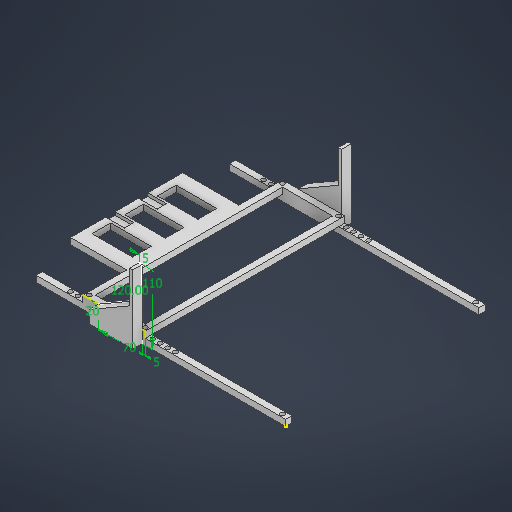
# Autodesk Inventor part: Pedal Box Mount V1
Saved by Autodesk Inventor 2027 (Build 310192000, 192)
## iProperties
Created: 2026-07-08
Part Number: Pedal Box Mount V1
Material: Generic
Document SubType Name: Modeling
Designer: W Ahmad
Density: 1 g/cm^3
Appearance: Default
Author: W Ahmad
Autodesk Inventor part; units mm, degrees
ref_plane "YZ Plane" through (0, 0, 0) normal (1, 0, 0) x (0, 1, 0)
ref_plane "XZ Plane" through (0, 0, 0) normal (0, 1, 0) x (-1, 0, 0)
ref_plane "XY Plane" through (0, 0, 0) normal (0, 0, 1) x (1, 0, 0)
sketch "Sketch1" plane through (0, 0, 0) normal (0, 1, 0) x (-1, 0, 0)
  line L0 (400, 160) -> (0, 160)
  line L1 (0, 160) -> (0, 150)
  line L2 (0, 150) -> (400, 150)
  line L3 (400, 150) -> (400, 160)
  line L4 (400, -150) -> (0, -150)
  line L5 (0, -150) -> (0, -160)
  line L6 (0, -160) -> (400, -160)
  line L7 (400, -160) -> (400, -150)
  line L8 (0, 150) -> (0, 0) construction
  line L9 (0, 0) -> (200, 0) construction
  circle A0 centre (350, 155) radius 3.5
  circle A1 centre (350, -155) radius 3.5
  circle A2 centre (338, 155) radius 3.5
  circle A3 centre (338, -155) radius 3.5
  circle A4 centre (326, 155) radius 3.5
  circle A5 centre (326, -155) radius 3.5
  circle A6 centre (314, 155) radius 3.5
  circle A7 centre (314, -155) radius 3.5
  circle A8 centre (302, 155) radius 3.5
  circle A9 centre (302, -155) radius 3.5
  circle A10 centre (290, 155) radius 3.5
  circle A11 centre (290, -155) radius 3.5
  circle A12 centre (278, 155) radius 3.5
  circle A13 centre (278, -155) radius 3.5
  circle A14 centre (266, 155) radius 3.5
  circle A15 centre (266, -155) radius 3.5
  circle A16 centre (254, 155) radius 3.5
  circle A17 centre (254, -155) radius 3.5
  circle A18 centre (242, 155) radius 3.5
  circle A19 centre (242, -155) radius 3.5
  circle A20 centre (230, 155) radius 3.5
  circle A21 centre (230, -155) radius 3.5
  circle A22 centre (218, 155) radius 3.5
  circle A23 centre (218, -155) radius 3.5
  circle A24 centre (206, 155) radius 3.5
  circle A25 centre (206, -155) radius 3.5
  circle A26 centre (194, 155) radius 3.5
  circle A27 centre (194, -155) radius 3.5
  circle A28 centre (182, 155) radius 3.5
  circle A29 centre (182, -155) radius 3.5
  circle A30 centre (10, 155) radius 3.5
  circle A31 centre (10, -155) radius 3.5
  point P0 (400, 155)
  point P1 (400, -155)
  point P2 (0, -155)
  point P3 (0, 155)
  dimension "d0" = 10
  dimension "d1" = 400
  dimension "d2" = 300
  dimension "d3" = 150
  dimension "d4" = 200
  dimension "d5" = 50
  dimension "d6" = 7
  dimension "d7" = 7
  dimension "d8" = 50
  dimension "d11" = 12
  dimension "d16" = 7
  dimension "d17" = 10
  dimension "d18" = 10
  dimension "d19" = 7
  constraints: 32 centre point, 20 end point, 4 horizontal alignment, 4 midpoint, 4 parallel, 3 horizontal, 3 perpendicular, 2 point on line, 1 coincident, 1 collinear, 1 vertical, 56 other
  measures "d0" distance of L2.end L0.start
  measures "d1" distance of L0.start L0.end
  measures "d2" distance between parallel lines of L4 L2
  measures "d3" distance of L1.end L8.end
  measures "d4" distance of L8.end L9.end
  measures "d5" distance from line of L3 A0.centre
  measures "d6" diameter of A0
  measures "d7" diameter of A1
  measures "d8" distance from line of A1.centre L7
  measures "d11" distance of A0.centre A2.centre
  measures "d16" diameter of A31
  measures "d17" distance from line of L5 A31.centre
  measures "d18" distance from line of L1 A30.centre
  measures "d19" diameter of A30
extrude "Extrusion1" add sketch "Sketch1" along normal blind 10
sketch "Sketch2" plane through (0, 10, 0) normal (0, 1, 0) x (1, 0, 0)
  line L0 (-325, -160) -> (-225, -160)
  line L1 (-225, -160) -> (-225, 160)
  line L2 (-225, 160) -> (-325, 160)
  line L3 (-325, 160) -> (-325, -160)
  line L4 (0, 160) -> (-400, 160) projected
  line L5 (-400, -160) -> (0, -160) projected
  line L6 (0, -150) -> (-400, -150) projected
  line L7 (-400, 150) -> (0, 150) projected
  line L8 (-315, -150) -> (-235, -150)
  line L9 (-235, -150) -> (-235, 150)
  line L10 (-235, 150) -> (-315, 150)
  line L11 (-315, 150) -> (-315, -150)
  line L12 (-325, -90) -> (-415, -90)
  line L13 (-415, -90) -> (-415, 90)
  line L14 (-415, 90) -> (-325, 90)
  line L15 (-325, 90) -> (-325, -90)
  line L16 (-403, -67.5) -> (-338, -67.5)
  line L17 (-338, -67.5) -> (-338, -37.5)
  line L18 (-338, -37.5) -> (-403, -37.5)
  line L19 (-403, -37.5) -> (-403, -67.5)
  line L20 (-403, -15) -> (-338, -15)
  line L21 (-338, -15) -> (-338, 15)
  line L22 (-338, 15) -> (-403, 15)
  line L23 (-403, 15) -> (-403, -15)
  line L24 (-403, 37.5) -> (-338, 37.5)
  line L25 (-338, 37.5) -> (-338, 67.5)
  line L26 (-338, 67.5) -> (-403, 67.5)
  line L27 (-403, 67.5) -> (-403, 37.5)
  circle A0 centre (-320, -155) radius 3.5
  line L28 (0, -160) -> (0, -150) projected
  circle A1 centre (-320, 155) radius 3.5
  line L29 (-400, 160) -> (-400, 150) projected
  circle A2 centre (-230, -155) radius 3.5
  circle A3 centre (-230, 155) radius 3.5
  point P0 (0, 0)
  point P1 (-325, 0)
  point P2 (0, -155)
  point P3 (-400, 155)
  dimension "d22" = 0
  dimension "d23" = 0
  dimension "d25" = 10
  dimension "d26" = 10
  dimension "d27" = 80
  dimension "d28" = 225
  dimension "d31" = 180
  dimension "d33" = 60
  dimension "d34" = 90
  dimension "d35" = 30
  dimension "d36" = 30
  dimension "d37" = 30
  dimension "d38" = 65
  dimension "d41" = 12
  dimension "d42" = 22.5
  dimension "d43" = 22.5
  dimension "d44" = 22.5
  dimension "d48" = 5
  dimension "d49" = 7
  dimension "d50" = 5
  dimension "d51" = 7
  dimension "d54" = 90
  constraints: 48 end point, 12 parallel, 7 horizontal, 6 perpendicular, 5 point on line, 4 centre point, 3 midpoint, 2 collinear, 2 horizontal alignment, 4 other
  measures "d22" distance between parallel lines of L4 L2
  measures "d23" distance between parallel lines of L5 L0
  measures "d25" distance between parallel lines of L11 L3
  measures "d26" distance between parallel lines of L1 L9
  measures "d27" distance of L8.start L8.end
  measures "d28" distance from line of point (0, 0) L1
  measures "d31" distance of L12.end L13.end
  measures "d33" distance between parallel lines of L12 L6
  measures "d34" distance of L13.end L14.end
  measures "d35" distance of L22.end L20.start
  measures "d36" distance of L26.end L24.start
  measures "d37" distance of L18.end L16.start
  measures "d38" distance of L20.start L20.end
  measures "d41" distance between parallel lines of L23 L13
  measures "d42" distance between parallel lines of L14 L26
  measures "d43" distance between parallel lines of L24 L22
  measures "d44" distance between parallel lines of L20 L18
  measures "d48" distance from line of A0.centre L3
  measures "d49" diameter of A0
  measures "d50" distance from line of A1.centre L3
  measures "d51" diameter of A1
  measures "d54" distance of A0.centre A2.centre
extrude "Extrusion3" add sketch "Sketch2" along normal blind 10 contours L3 L6 L1 L0 | L3 L7 L11 L6 | L6 L9 L7 L1 | L12 L13 L14 L3 | L7 L3 L2 L1
sketch "Sketch3" plane through (0, 20, 0) normal (0, 1, 0) x (1, 0, 0)
  line L0 (-415, 90) -> (-415, -90) projected
  line L1 (-415, -33.5) -> (-385, -33.5)
  line L2 (-385, -33.5) -> (-385, -18.5)
  line L3 (-385, -18.5) -> (-415, -18.5)
  line L4 (-415, -18.5) -> (-415, -33.5)
  line L5 (-415, 19) -> (-385, 19)
  line L6 (-385, 19) -> (-385, 34)
  line L7 (-385, 34) -> (-415, 34)
  line L8 (-415, 34) -> (-415, 19)
  line L9 (-403, 15) -> (-338, 15) projected
  line L10 (-403, -37.5) -> (-338, -37.5) projected
  point P0 (0, 0)
  dimension "d61" = 0
  dimension "d62" = 30
  dimension "d63" = 15
  dimension "d64" = 15
  dimension "d65" = 4
  dimension "d66" = 4
  constraints: 16 end point, 4 parallel, 2 horizontal, 2 perpendicular, 1 collinear, 1 point on line
  measures "d61" distance between parallel lines of L0 L8
  measures "d62" distance of L1.start L1.end
  measures "d63" distance of L1.end L2.end
  measures "d64" distance of L5.end L6.end
  measures "d65" distance between parallel lines of L5 L9
  measures "d66" distance between parallel lines of L1 L10
extrude "Extrusion4" cut sketch "Sketch3" against normal blind 5
sketch "Sketch4" plane through (-400, 0, 160) normal (0, 0, 1) x (1, 0, 0)
  line L0 (100, 0) -> (170, 0)
  line L1 (170, 0) -> (170, 110)
  line L2 (170, 110) -> (165, 110)
  line L3 (165, 110) -> (165, 57.5278)
  line L4 (100, 0) -> (100, 20)
  line L5 (75, 20) -> (175, 20) projected
  line L6 (165, 57.5278) -> (100, 20)
  line L7 (175, 10) -> (175, 20) projected
  point P0 (400, 0)
  dimension "d69" = 120
  dimension "d70" = 5
  dimension "d71" = 110
  dimension "d72" = 70
  dimension "d73" = 20
  dimension "d74" = 5
  constraints: 12 end point, 3 perpendicular, 1 horizontal, 1 point on line, 1 vertical
  measures "d69" angle of L3 L6
  measures "d70" distance of L1.end L2.end
  measures "d71" distance of L0.end L1.end
  measures "d72" distance of L0.start L0.end
  measures "d73" distance of L0.start L4.end
  measures "d74" distance between parallel lines of L7 L1
extrude "Extrusion5" add sketch "Sketch4" along normal blind 15
sketch "Sketch5" plane through (0, 0, -160) normal (0, 0, -1) x (-1, 0, 0)
  line L0 (300, 0) -> (230, 0) projected
  line L1 (300, 0) -> (230, 0)
  line L2 (230, 0) -> (230, 110)
  line L3 (230, 110) -> (235, 110)
  line L4 (235, 110) -> (235, 57.5278)
  line L5 (325, 20) -> (225, 20) projected
  line L6 (235, 57.5278) -> (300, 20)
  line L7 (300, 20) -> (300, 0)
  point P0 (0, 0)
  point P1 (230, 20)
  dimension "d83" = 110
  dimension "d84" = 120
  dimension "d85" = 5
  constraints: 12 end point, 3 perpendicular, 1 horizontal, 1 parallel
  measures "d83" distance of L0.end L2.end
  measures "d84" angle of L6 L4
  measures "d85" distance of L2.end L3.end
extrude "Extrusion6" add sketch "Sketch5" along normal blind 15
body "Solid1"
